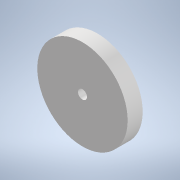
# Autodesk Inventor part: Pieza44
Saved by Autodesk Inventor 2022.2 (Build 262287000, 287)
## iProperties
Created: 2022-02-11
Part Number: Pieza44
Material: Genérico
Document SubType Name: Modeling
Designer: USUARIO
Density: 1 g/cm^3
Appearance: Valor por defecto
Author: USUARIO
Autodesk Inventor part; units mm, degrees
ref_plane "YZ Plane" through (0, 0, 0) normal (1, 0, 0) x (0, 1, 0)
ref_plane "XZ Plane" through (0, 0, 0) normal (0, 1, 0) x (-1, 0, 0)
ref_plane "XY Plane" through (0, 0, 0) normal (0, 0, 1) x (1, 0, 0)
sketch "Boceto1" plane through (0, 0, 0) normal (0, 0, 1) x (1, 0, 0)
  circle A0 centre (0, 0) radius 4.5
  circle A1 centre (0, 0) radius 45
  dimension "d0" = 9
  dimension "d1" = 90
  constraints: 2 centre point, 2 coincident
  measures "d0" diameter of A0
  measures "d1" diameter of A1
extrude "Extrusión1" add sketch "Boceto1" along normal blind 15
sketch "Boceto2" plane through (0, 0, 0) normal (0, 0, -1) x (-1, 0, 0)
  arc A0 (-6.9941, 2.7079) -> (-6.9941, -2.7079) centre (0, 0) ccw
  arc A1 (-33.0366, 17.7436) -> (-33.0366, -17.7436) centre (0, 0) ccw
  line L0 (-6.9941, 2.7079) -> (-33.0366, 17.7436)
  line L1 (-6.9941, -2.7079) -> (-33.0366, -17.7436)
  line L2 (-2.7079, -6.9941) -> (-17.7436, -33.0366)
  arc A2 (-17.7436, -33.0366) -> (17.7436, -33.0366) centre (0, 0) ccw
  line L3 (2.7079, -6.9941) -> (17.7436, -33.0366)
  arc A3 (-2.7079, -6.9941) -> (2.7079, -6.9941) centre (0, 0) ccw
  line L4 (6.9941, -2.7079) -> (33.0366, -17.7436)
  arc A4 (33.0366, -17.7436) -> (33.0366, 17.7436) centre (0, 0) ccw
  line L5 (6.9941, 2.7079) -> (33.0366, 17.7436)
  arc A5 (6.9941, -2.7079) -> (6.9941, 2.7079) centre (0, 0) ccw
  line L6 (2.7079, 6.9941) -> (17.7436, 33.0366)
  arc A6 (17.7436, 33.0366) -> (-17.7436, 33.0366) centre (0, 0) ccw
  line L7 (-2.7079, 6.9941) -> (-17.7436, 33.0366)
  arc A7 (2.7079, 6.9941) -> (-2.7079, 6.9941) centre (0, 0) ccw
  dimension "d4" = 15
  dimension "d5" = 75
  dimension "d13" = 360
  constraints: 16 end point, 16 point on circle, 8 centre point, 5 coincident, 41 other
  measures "d4" diameter of A0
  measures "d5" diameter of A1
extrude "Extrusión2" cut sketch "Boceto2" against normal through all
